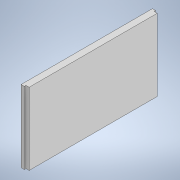
# Autodesk Inventor part: Lid
Saved by Autodesk Inventor 2020 (Build 240168000, 168)
## iProperties
Created: 2019-09-30
Part Number: Lid
Material: Generic
Document SubType Name: Modeling
Designer: bzs3334
Density: 1 g/cm^3
Appearance: Default
Author: bzs3334
Autodesk Inventor part; units mm, degrees
ref_plane "YZ Plane" through (0, 0, 0) normal (1, 0, 0) x (0, 1, 0)
ref_plane "XZ Plane" through (0, 0, 0) normal (0, 1, 0) x (-1, 0, 0)
ref_plane "XY Plane" through (0, 0, 0) normal (0, 0, 1) x (1, 0, 0)
sketch "Sketch1" plane through (0, 0, 0) normal (1, 0, 0) x (0, 1, 0)
  line L0 (22.5, 41) -> (-22.5, 41)
  line L1 (-22.5, 41) -> (-22.5, -41)
  line L2 (-22.5, -41) -> (22.5, -41)
  line L3 (22.5, -41) -> (22.5, 41)
  point P0 (0, 0)
  dimension "d0" = 82
  dimension "d1" = 41
  dimension "d2" = 45
  dimension "d3" = 22.5
  constraints: 8 end point, 2 parallel, 1 horizontal, 1 perpendicular
  measures "d0" distance of L2.end L0.start
  measures "d1" distance from line of L0 point (0, 0)
  measures "d2" distance of L0.start L0.end
  measures "d3" horizontal distance of L0.end point (0, 0)
extrude "Extrusion1" add sketch "Sketch1" along normal blind 2
sketch "Sketch2" plane through (2, 0, 0) normal (1, 0, 0) x (0, 0, -1)
  line L0 (41, 22.5) -> (-41, 22.5) projected
  line L1 (-41, -22.5) -> (41, -22.5) projected
  line L2 (-40, 22.5) -> (40, 22.5)
  line L3 (40, 22.5) -> (40, -22.5)
  line L4 (40, -22.5) -> (-40, -22.5)
  line L5 (-40, -22.5) -> (-40, 22.5)
  line L6 (-41, 22.5) -> (-41, -22.5) projected
  line L7 (41, -22.5) -> (41, 22.5) projected
  point P0 (0, 0)
  point P1 (-40, -22.5)
  dimension "d6" = 1
  dimension "d7" = 1
  constraints: 8 end point, 2 parallel, 2 point on line, 1 horizontal, 1 perpendicular
  measures "d6" distance between parallel lines of L6 L5
  measures "d7" distance between parallel lines of L3 L7
extrude "Extrusion2" add sketch "Sketch2" along normal blind 2 contours L3 L1 L5 L0
equation "\"d1\" = 0.5 * d0"
equation "\"d3\" = 0.5 * d2"
body "Solid1"
